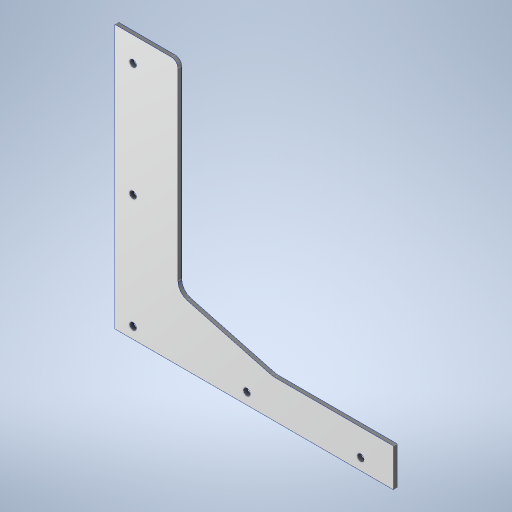
# Autodesk Inventor part: Door Stiffening Gusset
Saved by Autodesk Inventor 2024 (Build 280153000, 153)
## iProperties
Created: 2024-09-28
Part Number: Door Stiffening Gusset
Material: Generic
Document SubType Name: Modeling
Designer: Ishaan
Density: 1 g/cm^3
Appearance: Default
Author: Ishaan
Autodesk Inventor part; units mm, degrees
ref_plane "YZ Plane" through (0, 0, 0) normal (1, 0, 0) x (0, 1, 0)
ref_plane "XZ Plane" through (0, 0, 0) normal (0, 1, 0) x (-1, 0, 0)
ref_plane "XY Plane" through (0, 0, 0) normal (0, 0, 1) x (1, 0, 0)
sketch "Sketch1" plane through (0, 0, 0) normal (0, 0, 1) x (1, 0, 0)
  line L0 (110.25, -104.25) -> (-110.25, -104.25)
  line L1 (-110.25, -104.25) -> (-110.25, 104.25)
  line L2 (-110.25, 104.25) -> (110.25, 104.25)
  line L3 (110.25, 104.25) -> (110.25, -104.25)
  line L4 (110.25, -104.25) -> (-110.25, 104.25) construction
  line L5 (-110.25, -104.25) -> (110.25, 104.25) construction
  line L6 (110.25, -104.25) -> (-110.25, -104.25)
  line L7 (-110.25, -104.25) -> (-110.25, -74.25)
  line L8 (-110.25, -74.25) -> (110.25, -74.25)
  line L9 (110.25, -74.25) -> (110.25, -104.25)
  line L10 (-60.25, -74.25) -> (-60.25, 104.25)
  line L11 (-60.25, -54.1538) -> (14.75, -74.25)
  point P0 (0, 0)
  point P1 (110.25, -74.25)
  dimension "d101" = 220.5
  dimension "d102" = 208.5
  dimension "d103" = 30
  dimension "d105" = 165
  dimension "d106" = 50
  dimension "d107" = 75
  constraints: 24 end point, 5 point on line, 4 parallel, 3 perpendicular, 2 horizontal, 2 midpoint
  measures "d101" distance of L1.end L2.end
  measures "d102" distance of L0.end L1.end
  measures "d103" distance of L6.end L7.end
  measures "d105" angle of L8 L11
  measures "d106" distance between parallel lines of L1 L10
  measures "d107" distance from line of L11.end L10
extrude "Extrusion1" add sketch "Sketch1" along normal mid plane 3 contours L0 L1 L8 L3 | L1 L2 L10 L8 | L8 L10 L11
extrude "Extrusion2" cut sketch "Sketch1" along normal mid plane 2.9 contours L0 L1 L8 L3 | L1 L2 L10 L8 | L8 L10 L11
extrude "Extrusion3" add sketch "Sketch1" along normal mid plane 2.9 separate body contours L0 L1 L8 L3 | L1 L2 L10 L8 | L8 L10 L11
fillet "Fillet1" radius 10 6 edges at (-60.25, -54.1538, -1.475) (-60.25, -54.1538, 1.475) (14.75, -74.25, -1.475) (14.75, -74.25, 1.475) (-60.25, -54.1538, 0) (14.75, -74.25, 0)
fillet "Fillet2" radius 5 3 edges at (-60.25, 104.25, 1.475) (-60.25, 104.25, -1.475) (-60.25, 104.25, 0)
sketch "Sketch11" plane through (0, 0, 1.5) normal (0, 0, 1) x (1, 0, 0)
  line L0 (-110.25, 104.25) -> (-110.25, -104.25) construction
  line L1 (-110.25, -104.25) -> (110.25, -104.25) construction
  point P0 (0, 0)
  point P1 (-95.75, -95.25)
  point P2 (-95.75, -50.25)
  point P3 (-95.75, -5.25)
  point P4 (-95.75, 39.75)
  point P5 (-95.75, 84.75)
  point P6 (-50.75, -95.25)
  point P7 (-5.75, -95.25)
  point P8 (39.25, -95.25)
  point P9 (84.25, -95.25)
  dimension "d112" = 45
  dimension "d117" = 9
  dimension "d118" = 14.5
  dimension "d121" = 45
  constraints: 1 horizontal, 1 vertical, 8 other
  measures "d112" distance of point (-95.75, -95.25) point (-95.75, -50.25)
  measures "d117" distance from line of point (-95.75, -95.25) L1
  measures "d118" distance from line of point (-95.75, -95.25) L0
  measures "d121" distance of point (-95.75, -95.25) point (-50.75, -95.25)
hole "Hole6" at (-95.75, -95.25, 1.5) at (-95.75, -5.25, 1.5) at (-95.75, 84.75, 1.5) at (-5.75, -95.25, 1.5) at (84.25, -95.25, 1.5) direction (0, 0, -1) diameter 5.3 end through all bodies 1 2
